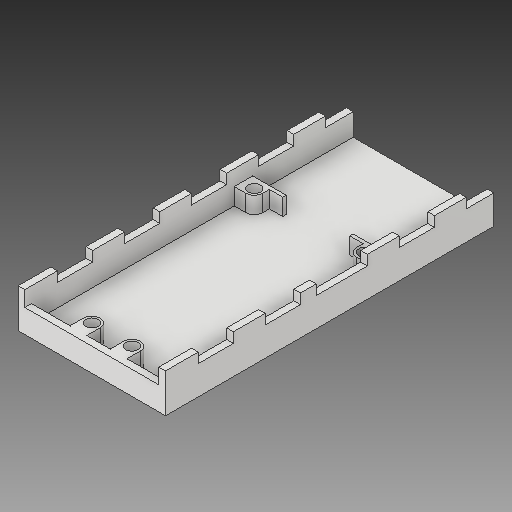
# Autodesk Inventor part: B6
Saved by Autodesk Inventor 2019.4 (Build 234330000, 330)
## iProperties
Created: 2019-05-28
Part Number: B6
Material: ABS Plastic
Document SubType Name: Modeling
Designer: Yichen Wang
Density: 1.06 g/cm^3
Appearance: Smooth - White
Mass: 13.26 g
Surface Area: 134.138 cm^2
Volume: 12.5094 cm^3
Description: VESC CASE BOTTOM
Author: Yichen Wang
Title: ESC CASE BOTTOM
Autodesk Inventor part; units mm, degrees
ref_plane "YZ Plane" through (0, 0, 0) normal (1, 0, 0) x (0, 1, 0)
ref_plane "XZ Plane" through (0, 0, 0) normal (0, 1, 0) x (-1, 0, 0)
ref_plane "XY Plane" through (0, 0, 0) normal (0, 0, 1) x (1, 0, 0)
sketch "Sketch1" plane through (0, 0, 0) normal (0, 1, 0) x (-1, 0, 0)
  line L0 (20, 32.5) -> (8.5, 32.5)
  line L1 (8.5, 32.5) -> (8.5, 28.5)
  arc A0 (3.5, 28.5) -> (8.5, 28.5) centre (6, 28.5) ccw
  line L2 (3.5, 28.5) -> (3.5, 32.5)
  line L3 (3.5, 32.5) -> (-3.5, 32.5)
  arc A1 (-8.5, 28.5) -> (-3.5, 28.5) centre (-6, 28.5) ccw
  line L4 (-8.5, 28.5) -> (-8.5, 32.5)
  line L5 (-8.5, 32.5) -> (-20, 32.5)
  line L6 (-20, 32.5) -> (-20, -28)
  line L7 (-20, -28) -> (-16.5, -28)
  arc A2 (-14, -30.5) -> (-16.5, -28) centre (-16.5, -30.5) ccw
  line L8 (-14, -30.5) -> (-14, -32.5)
  line L9 (-14, -32.5) -> (14, -32.5)
  line L10 (14, -32.5) -> (14, -30.5)
  arc A3 (16.5, -28) -> (14, -30.5) centre (16.5, -30.5) ccw
  line L11 (16.5, -28) -> (20, -28)
  line L12 (20, -28) -> (20, 32.5)
  line L13 (-21, 33.5) -> (21, 33.5)
  line L14 (21, 33.5) -> (21, -33.5)
  line L15 (21, -33.5) -> (-21, -33.5)
  line L16 (-21, -33.5) -> (-21, 33.5)
  line L17 (-3.5, 28.5) -> (-3.5, 32.5)
  circle A4 centre (-16.5, -30.5) radius 1.5
  circle A5 centre (6, 28.5) radius 1.5
  circle A6 centre (-6, 28.5) radius 1.5
  circle A7 centre (16.5, -30.5) radius 1.5
  line L18 (6, 28.5) -> (-6, 28.5) construction
  line L19 (16.5, -30.5) -> (-16.5, -30.5) construction
  line L20 (0, 28.5) -> (0, -30.5) construction
  line L21 (-21, 33.5) -> (21, -33.5) construction
  line L22 (-21, -33.5) -> (21, 33.5) construction
  line L23 (-3.5, 28.5) -> (-8.5, 28.5) construction
  line L24 (3.5, 28.5) -> (8.5, 28.5) construction
  line L25 (16.5, -28) -> (16.5, -30.5) construction
  line L26 (-16.5, -30.5) -> (-16.5, -28) construction
  point P0 (0, 0)
  point P1 (0, -1)
  point P2 (0, 0)
  dimension "d8" = 3
  dimension "d80" = 12
  dimension "d81" = 33
  dimension "d82" = 59
  dimension "d83" = 2.5
  dimension "d84" = 2.5
  dimension "d85" = 1
  dimension "d86" = 3
  dimension "d87" = 65
  dimension "d88" = 40
  dimension "d89" = 1
  dimension "d90" = 1
  dimension "d91" = 1
  dimension "d92" = 1
  dimension "d93" = 2.5
  dimension "d94" = 2.5
  dimension "d95" = 3
  dimension "d96" = 3
  constraints: 54 end point, 11 vertical, 9 horizontal, 8 centre point, 8 point on circle, 5 midpoint, 5 point on line, 4 concentric, 2 collinear, 1 parallel, 1 other
  measures "d8" diameter of A7
  measures "d80" distance of L18.start L18.end
  measures "d81" distance of L19.start L19.end
  measures "d82" distance of L20.start L20.end
  measures "d83" radius of A0
  measures "d84" radius of A1
  measures "d85" distance of point (0, 0) point (0, -1)
  measures "d86" diameter of A4
  measures "d87" distance between parallel lines of L9 L3
  measures "d88" distance between parallel lines of L6 L12
  measures "d89" distance between parallel lines of L12 L14
  measures "d90" distance between parallel lines of L9 L15
  measures "d91" distance between parallel lines of L5 L13
  measures "d92" distance between parallel lines of L16 L6
  measures "d93" radius of A3
  measures "d94" radius of A2
  measures "d95" diameter of A5
  measures "d96" diameter of A6
extrude "Extrusion1" add sketch "Sketch1" along normal blind 5
sketch "Sketch2" plane through (21, 0, -33.5) normal (0, 0, -1) x (-1, 0, 0)
  line L0 (42, 5) -> (0, 5) projected
  line L1 (31, 5) -> (21, 5)
  line L2 (21, 5) -> (21, 0)
  line L3 (21, 0) -> (31, 0)
  line L4 (31, 0) -> (31, 5)
  line L5 (21, 0) -> (11, 0)
  line L6 (11, 0) -> (11, 5)
  line L7 (11, 5) -> (21, 5)
  line L8 (21, 5) -> (21, 0)
  point P0 (21, 0)
  dimension "d11" = 10
  dimension "d12" = 10
  dimension "d13" = 0
  dimension "d14" = 0
  constraints: 16 end point, 4 parallel, 3 point on line, 2 horizontal, 2 perpendicular
  measures "d11" distance of L2.end L3.end
  measures "d12" distance of L5.start L5.end
  measures "d13" distance of point (21, 0) L2.end
  measures "d14" distance of L5.start point (21, 0)
extrude "Extrusion2" cut sketch "Sketch2" against normal up to surface (1 mm away)
sketch "Sketch3" plane through (0, 0, 0) normal (0, 1, 0) x (-1, 0, 0)
  line L0 (-21, -33.5) -> (-21, 33.5) projected
  line L1 (-21, 33.5) -> (21, 33.5)
  line L2 (21, 33.5) -> (21, -33.5)
  line L3 (21, -33.5) -> (-21, -33.5)
  line L4 (-21, -33.5) -> (-21, 33.5)
  point P0 (0, 0)
  constraints: 8 end point, 2 parallel, 1 horizontal, 1 perpendicular
extrude "Extrusion3" add sketch "Sketch3" against normal blind 1
sketch "Sketch5" plane through (16.5, 0, -30.5) normal (0, 1, 0) x (1, 0, 0)
  circle A0 centre (-10.5, -59) radius 1.5 projected
  point P0 (-10.5, -59)
  constraints: 1 coincident
hole "Hole1" at (6, 0, 28.5) direction (0, -1, 0) diameter 3.7 end through all both
sketch "Sketch6" plane through (16.5, 0, -30.5) normal (0, 1, 0) x (1, 0, 0)
  circle A0 centre (-22.5, -59) radius 1.5 projected
  point P0 (-22.5, -59)
  constraints: 1 coincident
hole "Hole2" at (-6, 0, 28.5) direction (0, -1, 0) diameter 3.7 end through all both
sketch "Sketch7" plane through (16.5, 0, -30.5) normal (0, 1, 0) x (1, 0, 0)
  circle A0 centre (-33, 0) radius 1.5 projected
  point P0 (-33, 0)
  constraints: 1 coincident
hole "Hole3" at (-16.5, 0, -30.5) direction (0, -1, 0) diameter 3.7 end through all both
sketch "Sketch8" plane through (16.5, 0, -30.5) normal (0, 1, 0) x (1, 0, 0)
  circle A0 centre (0, 0) radius 1.5 projected
  constraints: 1 coincident
hole "Hole4" at (16.5, 0, -30.5) direction (0, -1, 0) diameter 3.7 end through all both
sketch "Sketch4" plane through (21, 5, -33.5) normal (0, 0, -1) x (-1, 0, 0)
  line L0 (42, 0) -> (42, -6) projected
  line L1 (42, -6) -> (0, -6) projected
  line L2 (42, 0) -> (0, 0)
  line L3 (0, 0) -> (0, -6)
  line L4 (0, -6) -> (42, -6)
  line L5 (42, -6) -> (42, 0)
  line L6 (31, 0) -> (42, 0) projected
  line L7 (41, 0) -> (1, 0)
  line L8 (1, 0) -> (1, -5)
  line L9 (1, -5) -> (41, -5)
  line L10 (41, -5) -> (41, 0)
  point P0 (21, -5)
  dimension "d56" = 1
  dimension "d57" = 1
  dimension "d58" = 1
  constraints: 16 end point, 4 parallel, 2 horizontal, 2 perpendicular, 1 point on line
  measures "d56" distance between parallel lines of L1 L9
  measures "d57" distance between parallel lines of L3 L8
  measures "d58" distance between parallel lines of L0 L10
extrude "Extrusion4" add sketch "Sketch4" along normal blind 30 contours L0 L1 L3 L2 L8 L9 L10
thicken "Thicken1" operation add thickness 1 both sides no extend neighbours yes toward (-1, 0, 0) faces at (-21, 1.3333, -31.1667) (7, 1.3333, 33.5) (21, 1, 1.1667) (1.8524, -1, -10.34)
sketch "Sketch9" plane through (0, 5, 0) normal (0, 1, 0) x (1, 0, 0)
  line L0 (22, -34.5) -> (22, 63.5) projected
  line L1 (22, -34.5) -> (20, -34.5)
  line L2 (20, -34.5) -> (20, -24.75)
  line L3 (20, -24.75) -> (22, -24.75)
  line L4 (22, -24.75) -> (22, -34.5)
  line L5 (20, -14.25) -> (22, -14.25)
  line L6 (22, -14.25) -> (22, -4.75)
  line L7 (22, -4.75) -> (20, -4.75)
  line L8 (20, -4.75) -> (20, -14.25)
  line L9 (20, 5.75) -> (22, 5.75)
  line L10 (22, 5.75) -> (22, 15.25)
  line L11 (22, 15.25) -> (20, 15.25)
  line L12 (20, 15.25) -> (20, 5.75)
  line L13 (20, 25.75) -> (22, 25.75)
  line L14 (22, 25.75) -> (22, 35.25)
  line L15 (22, 35.25) -> (20, 35.25)
  line L16 (20, 35.25) -> (20, 25.75)
  line L17 (20, 45.75) -> (22, 45.75)
  line L18 (22, 45.75) -> (22, 55.25)
  line L19 (22, 55.25) -> (20, 55.25)
  line L20 (20, 55.25) -> (20, 45.75)
  point P0 (0, 0)
  dimension "d63" = 9.75
  dimension "d64" = 10.5
  dimension "d65" = 2
  dimension "d66" = 9.5
  dimension "d67" = 10.5
  dimension "d68" = 9.5
  dimension "d69" = 10.5
  dimension "d70" = 9.5
  dimension "d71" = 10.5
  dimension "d72" = 9.5
  constraints: 40 end point, 10 parallel, 6 point on line, 5 horizontal, 5 perpendicular, 2 collinear
  measures "d63" distance of L1.end L2.end
  measures "d64" distance of L5.start L2.end
  measures "d65" distance of L0.start L1.end
  measures "d66" distance of L7.end L5.start
  measures "d67" distance of L7.end L9.start
  measures "d68" distance of L11.end L9.start
  measures "d69" distance of L13.start L11.end
  measures "d70" distance of L15.end L13.start
  measures "d71" distance of L15.end L17.start
  measures "d72" distance of L19.end L17.start
extrude "Extrusion5" add sketch "Sketch9" along normal blind 3
mirror "Mirror1" about plane through (0, 0, 0) normal (1, 0, 0) of "Extrusion5"
sketch "Sketch10" plane through (-22, -2, -63.5) normal (-1, 0, 0) x (0, 0, 1)
  line L0 (17.75, 7) -> (28.25, 7) projected
  line L1 (53, 7) -> (44, 7)
  line L2 (44, 7) -> (44, 14)
  line L3 (44, 14) -> (53, 14)
  line L4 (53, 14) -> (53, 7)
  point P0 (63.5, 2)
  point P1 (30, 7)
  dimension "d75" = 14
  dimension "d76" = 7
  dimension "d77" = 9
  constraints: 8 end point, 2 parallel, 1 horizontal, 1 perpendicular, 1 point on line
  measures "d75" distance from line of point (30, 7) L2
  measures "d76" distance of L3.end L1.start
  measures "d77" distance of L2.end L3.end
extrude "Extrusion6" cut sketch "Sketch10" against normal up to surface (2 mm away) from surface at -42
thicken "Thicken2" operation add thickness 1.6 both sides no extend neighbours yes toward (0, 1, 0) faces at (20.6667, 8, 31.25)
thicken "Thicken3" operation add thickness 1.6 both sides no extend neighbours yes toward (0, 1, 0) faces at (20.6667, 5, 21.25)
thicken "Thicken4" operation add thickness 1.6 both sides no extend neighbours yes toward (0, 1, 0) faces at (21.3333, 8, 11.0833)
thicken "Thicken5" operation add thickness 1.6 both sides no extend neighbours yes toward (0, 1, 0) faces at (21.3333, 5, -2.25)
thicken "Thicken6" operation add thickness 1.6 both sides no extend neighbours yes toward (0, 1, 0) faces at (20.6667, 8, -8.9167)
thicken "Thicken7" operation add thickness 1.6 both sides no extend neighbours yes toward (0, 1, 0) faces at (21.3333, 5, -15.5833)
thicken "Thicken8" operation add thickness 1.6 both sides no extend neighbours no toward (0, 1, 0) faces at (20.6667, 8, -32.0833)
thicken "Thicken9" operation add thickness 1.6 both sides no extend neighbours no toward (0, 1, 0) faces at (20.6667, 5, -42.25)
thicken "Thicken10" operation add thickness 1.6 both sides no extend neighbours no toward (0, 1, 0) faces at (20.6667, 8, -52.0833)
thicken "Thicken11" operation add thickness 1.6 both sides no extend neighbours no toward (0, 1, 0) faces at (20.6667, 5, -58)
thicken "Thicken12" operation add thickness 1.6 both sides no extend neighbours no toward (0, 1, 0) faces at (-20.6667, 8, 31.25)
thicken "Thicken13" operation add thickness 1.6 both sides no extend neighbours no toward (0, 1, 0) faces at (-20.6667, 5, 21.25)
thicken "Thicken14" operation add thickness 1.6 both sides no extend neighbours no toward (0, 1, 0) faces at (-21.3333, 8, 11.0833)
thicken "Thicken15" operation add thickness 1.6 both sides no extend neighbours no toward (0, 1, 0) faces at (-21.3333, 5, -2.25)
thicken "Thicken16" operation add thickness 1.6 both sides no extend neighbours no toward (0, 1, 0) faces at (-20.6667, 8, -12.0833)
thicken "Thicken17" operation add thickness 1.6 both sides no extend neighbours no toward (0, 1, 0) faces at (-21.3333, 5, -18.75)
thicken "Thicken18" operation add thickness 1.6 both sides no extend neighbours no toward (0, 1, 0) faces at (-20.6667, 8, -32.0833)
thicken "Thicken19" operation add thickness 1.6 both sides no extend neighbours no toward (0, 1, 0) faces at (-21.3333, 5, -38.75)
thicken "Thicken20" operation add thickness 1.6 both sides no extend neighbours no toward (0, 1, 0) faces at (-20.6667, 8, -52.0833)
thicken "Thicken21" operation add thickness 1.6 both sides no extend neighbours no toward (0, 1, 0) faces at (-21.3333, 5, -58)
equation "\"d67\" = d64"
equation "\"d68\" = d66"
equation "\"d69\" = d64"
equation "\"d70\" = d68"
equation "\"d71\" = d69"
equation "\"d72\" = d66"
body "Solid1"
